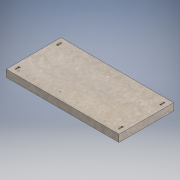
# Autodesk Inventor part: A soffit
Saved by Autodesk Inventor 2022.2 (Build 262287010, 287A)
## iProperties
Created: 2022-01-21
Part Number: A soffit
Material: Limestone
Document SubType Name: Modeling
Designer: awelt
Mass: 139091 g
Surface Area: 16952.5 cm^2
Volume: 53496.5 cm^3
Density: 2.6 g/cm^3
Appearance: Kasota Gray
Author: awelt
Autodesk Inventor part; units mm, degrees
ref_plane "YZ Plane" through (0, 0, 0) normal (1, 0, 0) x (0, 1, 0)
ref_plane "XZ Plane" through (0, 0, 0) normal (0, 1, 0) x (-1, 0, 0)
ref_plane "XY Plane" through (0, 0, 0) normal (0, 0, 1) x (1, 0, 0)
sketch "Bolt" plane through (0, 0, 0) normal (0, 0, 1) x (1, 0, 0)
  line L0 (25.0072, -4.4715) -> (29.7779, -8.6)
  line L1 (-7.366, -4.2392) -> (24.384, -4.2392)
  arc A0 (25.0072, -4.4715) -> (24.384, -4.2392) centre (24.384, -5.1917) ccw
  arc A1 (32.8161, -7.341) -> (33.3155, 0.6503) centre (-19.0704, -0.0877) ccw
  arc A2 (29.6829, -8.5178) -> (32.8161, -7.341) centre (30.9295, -7.0773) ccw
  line L2 (-7.366, -4.2392) -> (-7.366, 0.6503)
  line L3 (-7.366, 5.5398) -> (-7.366, 0.6503)
  line L4 (-7.366, 5.5398) -> (24.384, 5.5398)
  arc A3 (24.384, 5.5398) -> (25.0072, 5.772) centre (24.384, 6.4923) ccw
  line L5 (25.0072, 5.772) -> (29.7779, 9.9005)
  arc A4 (32.8161, 8.6415) -> (29.6829, 9.8183) centre (30.9295, 8.3778) ccw
  arc A5 (33.3155, 0.6503) -> (32.8161, 8.6415) centre (-19.0704, 1.3882) ccw
  dimension "d2" = 1203.325
sketch "Block2" plane through (0, 0, 0) normal (0, 0, 1) x (1, 0, 0)
  line L0 (55.9218, 83.1733) -> (60.0503, 87.944)
  line L1 (55.6895, 50.8) -> (55.6895, 82.55)
  arc A0 (55.9218, 83.1733) -> (55.6895, 82.55) centre (56.642, 82.55) ccw
  arc A1 (58.7912, 90.9822) -> (50.8, 91.4815) centre (51.5379, 39.0956) ccw
  arc A2 (59.968, 87.8489) -> (58.7912, 90.9822) centre (58.5275, 89.0955) ccw
  line L2 (55.6895, 50.8) -> (50.8, 50.8)
  line L3 (45.9105, 50.8) -> (50.8, 50.8)
  line L4 (45.9105, 50.8) -> (45.9105, 82.55)
  arc A3 (45.9105, 82.55) -> (45.6782, 83.1733) centre (44.958, 82.55) ccw
  line L5 (45.6782, 83.1733) -> (41.5497, 87.944)
  arc A4 (42.8088, 90.9822) -> (41.632, 87.8489) centre (43.0725, 89.0955) ccw
  arc A5 (50.8, 91.4815) -> (42.8088, 90.9822) centre (50.0621, 39.0956) ccw
  point P0 (50.8, 50.8)
  dimension "d2" = 1203.325
sketch "Block3" plane through (0, 0, 0) normal (0, 0, 1) x (1, 0, 0)
  line L0 (958.063, 109.0167) -> (953.9345, 104.246)
  line L1 (958.2953, 141.3899) -> (958.2953, 109.6399)
  arc A0 (958.063, 109.0167) -> (958.2953, 109.6399) centre (957.3428, 109.6399) ccw
  arc A1 (955.1935, 101.2078) -> (963.1848, 100.7084) centre (962.4468, 153.0943) ccw
  arc A2 (954.0168, 104.341) -> (955.1935, 101.2078) centre (955.4573, 103.0944) ccw
  line L2 (958.2953, 141.3899) -> (963.1848, 141.3899)
  line L3 (968.0743, 141.3899) -> (963.1848, 141.3899)
  line L4 (968.0743, 141.3899) -> (968.0743, 109.6399)
  arc A3 (968.0743, 109.6399) -> (968.3065, 109.0167) centre (969.0268, 109.6399) ccw
  line L5 (968.3065, 109.0167) -> (972.435, 104.246)
  arc A4 (971.176, 101.2078) -> (972.3528, 104.341) centre (970.9123, 103.0944) ccw
  arc A5 (963.1848, 100.7084) -> (971.176, 101.2078) centre (963.9227, 153.0943) ccw
  point P0 (963.1848, 141.3899)
  dimension "d2" = 1203.325
sketch "Sketch1" plane through (0, 0, 0) normal (1, 0, 0) x (0, 1, 0)
  line L0 (0, 0) -> (50.8, 0)
  line L1 (50.8, 0) -> (50.8, 584.2)
  line L2 (50.8, 584.2) -> (0, 584.2)
  line L3 (0, 584.2) -> (0, 0) construction
  line L4 (0, 584.2) -> (-25.4, 584.2)
  line L5 (-25.4, 584.2) -> (-25.4, 0)
  line L6 (-25.4, 0) -> (0, 0)
  dimension "d0" = 50.8
  dimension "d1" = 584.2
  dimension "d5" = 25.4
  constraints: 14 end point, 3 horizontal, 2 parallel, 2 perpendicular
  measures "d0" distance of L2.end L1.end
  measures "d1" distance of L1.end L0.end
  measures "d5" distance of L2.end L4.end
extrude "Extrusion1" add sketch "Sketch1" along normal blind 1203.325
sketch "Sketch2" plane through (0, 50.8, 584.2) normal (0, 1, 0) x (1, 0, 0)
  line L0 (0, 584.2) -> (0, 0) projected
  line L1 (0, 0) -> (1203.325, 0) projected
  line L2 (1203.325, 584.2) -> (1203.325, 0) projected
  line L3 (0, 584.2) -> (1203.325, 584.2) projected
  line L4 (1152.525, 533.4) -> (1152.525, 50.8) construction
  line L5 (1152.525, 50.8) -> (50.8, 50.8) construction
  line L6 (50.8, 50.8) -> (50.8, 533.4) construction
  line L7 (50.8, 533.4) -> (1152.525, 533.4) construction
  line L8 (55.9218, 83.1733) -> (60.0503, 87.944)
  line L9 (55.6895, 50.8) -> (55.6895, 82.55)
  arc A0 (55.9218, 83.1733) -> (55.6895, 82.55) centre (56.642, 82.55) ccw
  arc A1 (58.7912, 90.9822) -> (50.8, 91.4815) centre (51.5379, 39.0956) ccw
  arc A2 (59.968, 87.8489) -> (58.7912, 90.9822) centre (58.5275, 89.0955) ccw
  line L10 (55.6895, 50.8) -> (50.8, 50.8)
  line L11 (45.9105, 50.8) -> (50.8, 50.8)
  line L12 (45.9105, 50.8) -> (45.9105, 82.55)
  arc A3 (45.9105, 82.55) -> (45.6782, 83.1733) centre (44.958, 82.55) ccw
  line L13 (45.6782, 83.1733) -> (41.5497, 87.944)
  arc A4 (42.8088, 90.9822) -> (41.632, 87.8489) centre (43.0725, 89.0955) ccw
  arc A5 (50.8, 91.4815) -> (42.8088, 90.9822) centre (50.0621, 39.0956) ccw
  line L14 (1157.6468, 83.1733) -> (1161.7753, 87.944)
  line L15 (1157.4145, 50.8) -> (1157.4145, 82.55)
  arc A6 (1157.6468, 83.1733) -> (1157.4145, 82.55) centre (1158.367, 82.55) ccw
  arc A7 (1160.5162, 90.9822) -> (1152.525, 91.4815) centre (1153.2629, 39.0956) ccw
  arc A8 (1161.693, 87.8489) -> (1160.5162, 90.9822) centre (1160.2525, 89.0955) ccw
  line L16 (1157.4145, 50.8) -> (1152.525, 50.8)
  line L17 (1147.6355, 50.8) -> (1152.525, 50.8)
  line L18 (1147.6355, 50.8) -> (1147.6355, 82.55)
  arc A9 (1147.6355, 82.55) -> (1147.4032, 83.1733) centre (1146.683, 82.55) ccw
  line L19 (1147.4032, 83.1733) -> (1143.2747, 87.944)
  arc A10 (1144.5338, 90.9822) -> (1143.357, 87.8489) centre (1144.7975, 89.0955) ccw
  arc A11 (1152.525, 91.4815) -> (1144.5338, 90.9822) centre (1151.7871, 39.0956) ccw
  line L20 (1147.4032, 501.0267) -> (1143.2747, 496.256)
  line L21 (1147.6355, 533.4) -> (1147.6355, 501.65)
  arc A12 (1147.4032, 501.0267) -> (1147.6355, 501.65) centre (1146.683, 501.65) ccw
  arc A13 (1144.5338, 493.2178) -> (1152.525, 492.7185) centre (1151.7871, 545.1044) ccw
  arc A14 (1143.357, 496.3511) -> (1144.5338, 493.2178) centre (1144.7975, 495.1045) ccw
  line L22 (1147.6355, 533.4) -> (1152.525, 533.4)
  line L23 (1157.4145, 533.4) -> (1152.525, 533.4)
  line L24 (1157.4145, 533.4) -> (1157.4145, 501.65)
  arc A15 (1157.4145, 501.65) -> (1157.6468, 501.0267) centre (1158.367, 501.65) ccw
  line L25 (1157.6468, 501.0267) -> (1161.7753, 496.256)
  arc A16 (1160.5162, 493.2178) -> (1161.693, 496.3511) centre (1160.2525, 495.1045) ccw
  arc A17 (1152.525, 492.7185) -> (1160.5162, 493.2178) centre (1153.2629, 545.1044) ccw
  line L26 (45.6782, 501.0267) -> (41.5497, 496.256)
  line L27 (45.9105, 533.4) -> (45.9105, 501.65)
  arc A18 (45.6782, 501.0267) -> (45.9105, 501.65) centre (44.958, 501.65) ccw
  arc A19 (42.8088, 493.2178) -> (50.8, 492.7185) centre (50.0621, 545.1044) ccw
  arc A20 (41.632, 496.3511) -> (42.8088, 493.2178) centre (43.0725, 495.1045) ccw
  line L28 (45.9105, 533.4) -> (50.8, 533.4)
  line L29 (55.6895, 533.4) -> (50.8, 533.4)
  line L30 (55.6895, 533.4) -> (55.6895, 501.65)
  arc A21 (55.6895, 501.65) -> (55.9218, 501.0267) centre (56.642, 501.65) ccw
  line L31 (55.9218, 501.0267) -> (60.0503, 496.256)
  arc A22 (58.7912, 493.2178) -> (59.968, 496.3511) centre (58.5275, 495.1045) ccw
  arc A23 (50.8, 492.7185) -> (58.7912, 493.2178) centre (51.5379, 545.1044) ccw
  point P0 (1157.6468, 83.1733)
  point P1 (1161.693, 87.8489)
  point P2 (1160.5162, 90.9822)
  point P3 (1152.525, 91.4815)
  point P4 (1144.5338, 90.9822)
  point P5 (1143.357, 87.8489)
  point P6 (1147.4032, 83.1733)
  point P7 (1147.6355, 50.8)
  point P8 (1152.525, 50.8)
  point P9 (1157.4145, 50.8)
  point P10 (55.6895, 82.55)
  point P11 (55.9218, 83.1733)
  point P12 (59.968, 87.8489)
  point P13 (58.7912, 90.9822)
  point P14 (50.8, 91.4815)
  point P15 (42.8088, 90.9822)
  point P16 (41.632, 87.8489)
  point P17 (45.6782, 83.1733)
  point P18 (45.9105, 82.55)
  point P19 (45.9105, 50.8)
  point P20 (50.8, 50.8)
  point P21 (55.6895, 50.8)
  point P22 (45.9105, 501.65)
  point P23 (45.6782, 501.0267)
  point P24 (41.632, 496.3511)
  point P25 (42.8088, 493.2178)
  point P26 (50.8, 492.7185)
  point P27 (58.7912, 493.2178)
  point P28 (59.968, 496.3511)
  point P29 (55.9218, 501.0267)
  point P30 (55.6895, 501.65)
  point P31 (55.6895, 533.4)
  point P32 (50.8, 533.4)
  point P33 (45.9105, 533.4)
  point P34 (1147.6355, 501.65)
  point P35 (1147.4032, 501.0267)
  point P36 (1143.357, 496.3511)
  point P37 (1144.5338, 493.2178)
  point P38 (1161.693, 496.3511)
  point P39 (1157.6468, 501.0267)
  point P40 (1152.525, 533.4)
  point P41 (1147.6355, 533.4)
  dimension "d2" = 1203.325
  dimension "d4" = 50.8
  constraints: 8 end point, 7 other
  measures "d4" distance between parallel lines of L3 L7
revolve "Revolution1" cut sketch "Sketch2" angle 90 about axis through (1152.525, 50.8, 533.4) along (-1, 0, 0) contours A0 L9 L10 L11 L12 A3 L13 A4 A5 A1 A2 L8 | A6 L15 L16 L17 L18 A9 L19 A10 A11 A7 A8 L14
revolve "Revolution2" cut sketch "Sketch2" angle 90 about axis through (50.8, 50.8, 50.8) along (1, 0, 0) contours A12 L21 L22 L23 L24 A15 L25 A16 A17 A13 A14 L20 | A18 L27 L28 L29 L30 A21 L31 A22 A23 A19 A20 L26
sketch "Sketch3" plane through (45.9105, 50.8, 50.8) normal (0, 0, 1) x (1, 0, 0)
  line L0 (4.8895, 0) -> (4.8895, -40.6815)
  line L1 (1106.6145, 0) -> (1106.6145, -40.6815)
  line L2 (1101.4927, -32.3733) -> (1097.3642, -37.144)
  line L3 (1101.725, 0) -> (1101.725, -31.75)
  arc A0 (1101.4927, -32.3733) -> (1101.725, -31.75) centre (1100.7725, -31.75) ccw
  arc A1 (1098.6233, -40.1822) -> (1106.6145, -40.6815) centre (1105.8766, 11.7044) ccw
  arc A2 (1097.4465, -37.0489) -> (1098.6233, -40.1822) centre (1098.887, -38.2955) ccw
  line L4 (1101.725, 0) -> (1106.6145, 0)
  line L5 (1111.504, 0) -> (1106.6145, 0)
  line L6 (1111.504, 0) -> (1111.504, -31.75)
  arc A3 (1111.504, -31.75) -> (1111.7363, -32.3733) centre (1112.4565, -31.75) ccw
  line L7 (1111.7363, -32.3733) -> (1115.8648, -37.144)
  arc A4 (1114.6057, -40.1822) -> (1115.7825, -37.0489) centre (1114.342, -38.2955) ccw
  arc A5 (1106.6145, -40.6815) -> (1114.6057, -40.1822) centre (1107.3524, 11.7044) ccw
  line L8 (-0.2323, -32.3733) -> (-4.3608, -37.144)
  line L9 (0, 0) -> (0, -31.75)
  arc A6 (-0.2323, -32.3733) -> (0, -31.75) centre (-0.9525, -31.75) ccw
  arc A7 (-3.1017, -40.1822) -> (4.8895, -40.6815) centre (4.1516, 11.7044) ccw
  arc A8 (-4.2785, -37.0489) -> (-3.1017, -40.1822) centre (-2.838, -38.2955) ccw
  line L10 (0, 0) -> (4.8895, 0)
  line L11 (9.779, 0) -> (4.8895, 0)
  line L12 (9.779, 0) -> (9.779, -31.75)
  arc A9 (9.779, -31.75) -> (10.0113, -32.3733) centre (10.7315, -31.75) ccw
  line L13 (10.0113, -32.3733) -> (14.1398, -37.144)
  arc A10 (12.8807, -40.1822) -> (14.0575, -37.0489) centre (12.617, -38.2955) ccw
  arc A11 (4.8895, -40.6815) -> (12.8807, -40.1822) centre (5.6274, 11.7044) ccw
  point P0 (-45.9105, -50.8)
  point P1 (4.8895, 0)
  point P2 (1106.6145, 0)
  point P3 (10.0113, -32.3733)
  point P4 (9.779, -31.75)
  point P5 (9.779, 0)
  point P6 (4.8895, 0)
  point P7 (4.8895, -40.6815)
  point P8 (12.8807, -40.1822)
  point P9 (14.0575, -37.0489)
  point P10 (1111.7363, -32.3733)
  point P11 (1111.504, -31.75)
  point P12 (1111.504, 0)
  point P13 (1106.6145, 0)
  point P14 (1106.6145, -40.6815)
  point P15 (1114.6057, -40.1822)
  point P16 (1115.7825, -37.0489)
  dimension "d2" = 1203.325
  constraints: 4 end point, 2 vertical, 6 other
revolve "Revolution3" cut sketch "Sketch3" angle 360 about axis through (50.8, 50.8, 50.8) along (0, -1, 0) contours L11 L12 A9 L13 A10 A11 L0
revolve "Revolution4" cut sketch "Sketch3" angle 360 about axis through (1152.525, 50.8, 50.8) along (0, -1, 0) contours L5 L6 A3 L7 A4 A5 L1
sketch "Sketch4" plane through (1157.4145, 50.8, 533.4) normal (0, 0, -1) x (-1, 0, 0)
  line L0 (1106.6145, 0) -> (1106.6145, -40.6815)
  line L1 (4.8895, 0) -> (4.8895, -40.6815)
  line L2 (-0.2323, -32.3733) -> (-4.3608, -37.144)
  line L3 (0, 0) -> (0, -31.75)
  arc A0 (-0.2323, -32.3733) -> (0, -31.75) centre (-0.9525, -31.75) ccw
  arc A1 (-3.1017, -40.1822) -> (4.8895, -40.6815) centre (4.1516, 11.7044) ccw
  arc A2 (-4.2785, -37.0489) -> (-3.1017, -40.1822) centre (-2.838, -38.2955) ccw
  line L4 (0, 0) -> (4.8895, 0)
  line L5 (9.779, 0) -> (4.8895, 0)
  line L6 (9.779, 0) -> (9.779, -31.75)
  arc A3 (9.779, -31.75) -> (10.0113, -32.3733) centre (10.7315, -31.75) ccw
  line L7 (10.0113, -32.3733) -> (14.1398, -37.144)
  arc A4 (12.8807, -40.1822) -> (14.0575, -37.0489) centre (12.617, -38.2955) ccw
  arc A5 (4.8895, -40.6815) -> (12.8807, -40.1822) centre (5.6274, 11.7044) ccw
  line L8 (1101.4927, -32.3733) -> (1097.3642, -37.144)
  line L9 (1101.725, 0) -> (1101.725, -31.75)
  arc A6 (1101.4927, -32.3733) -> (1101.725, -31.75) centre (1100.7725, -31.75) ccw
  arc A7 (1098.6233, -40.1822) -> (1106.6145, -40.6815) centre (1105.8766, 11.7044) ccw
  arc A8 (1097.4465, -37.0489) -> (1098.6233, -40.1822) centre (1098.887, -38.2955) ccw
  line L10 (1101.725, 0) -> (1106.6145, 0)
  line L11 (1111.504, 0) -> (1106.6145, 0)
  line L12 (1111.504, 0) -> (1111.504, -31.75)
  arc A9 (1111.504, -31.75) -> (1111.7363, -32.3733) centre (1112.4565, -31.75) ccw
  line L13 (1111.7363, -32.3733) -> (1115.8648, -37.144)
  arc A10 (1114.6057, -40.1822) -> (1115.7825, -37.0489) centre (1114.342, -38.2955) ccw
  arc A11 (1106.6145, -40.6815) -> (1114.6057, -40.1822) centre (1107.3524, 11.7044) ccw
  point P0 (1157.4145, -50.8)
  point P1 (1106.6145, 0)
  point P2 (4.8895, 0)
  point P3 (10.0113, -32.3733)
  point P4 (9.779, -31.75)
  point P5 (9.779, 0)
  point P6 (4.8895, 0)
  point P7 (4.8895, -40.6815)
  point P8 (12.8807, -40.1822)
  point P9 (14.0575, -37.0489)
  point P10 (1111.7363, -32.3733)
  point P11 (1111.504, -31.75)
  point P12 (1111.504, 0)
  point P13 (1106.6145, -40.6815)
  point P14 (1114.6057, -40.1822)
  point P15 (1115.7825, -37.0489)
  dimension "d2" = 1203.325
  constraints: 4 end point, 2 vertical, 6 other
revolve "Revolution5" cut sketch "Sketch4" angle 360 about axis through (1152.525, 50.8, 533.4) along (0, -1, 0) contours L5 L6 A3 L7 A4 A5 L1
revolve "Revolution6" cut sketch "Sketch4" angle 360 about axis through (50.8, 50.8, 533.4) along (0, -1, 0) contours L11 L12 A9 L13 A10 A11 L0
body "Solid1"
